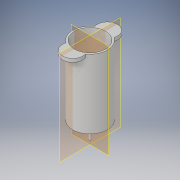
# Autodesk Inventor part: ReducedLargeSyrgine
Saved by Autodesk Inventor 2018 (Build 220112000, 112)
## iProperties
Created: 2020-03-29
Part Number: ReducedLargeSyrgine
Material: Generic
Document SubType Name: Modeling
Designer: Jesse R-B
Density: 1 g/cm^3
Appearance: Default
Author: Jesse R-B
Autodesk Inventor part; units mm, degrees
ref_plane "XZ Plane" through (0, 0, 0) normal (0, 1, 0) x (-1, 0, 0)
sketch "Sketch1" plane through (0, 0, 0) normal (0, 1, 0) x (-1, 0, 0)
  circle A0 centre (0, 0) radius 25.4
  dimension "d0" = 50.8
  constraints: 1 centre point, 1 coincident
  measures "d0" diameter of A0
extrude "Extrusion1" add sketch "Sketch1" along normal blind 101.6
sketch "Sketch2" plane through (0, 101.6, 0) normal (0, 1, 0) x (1, 0, 0)
  circle A0 centre (0, 0) radius 25.4 projected
  circle A1 centre (0, -25.4) radius 14.9225
  circle A2 centre (0, 25.4) radius 14.9225
  dimension "d3" = 29.845
  dimension "d4" = 29.845
  constraints: 2 centre point, 2 point on circle
  measures "d3" diameter of A1
  measures "d4" diameter of A2
extrude "Extrusion2" add sketch "Sketch2" against normal blind 5.08
sketch "Sketch3" plane through (0, 101.6, 0) normal (0, 1, 0) x (1, 0, 0)
  circle A0 centre (0, 0) radius 22.86
  dimension "d7" = 45.72
  constraints: 1 centre point, 1 coincident
  measures "d7" diameter of A0
extrude "Extrusion3" cut sketch "Sketch3" against normal blind 195.072
sketch "Sketch4" plane through (0, 0, 0) normal (0, -1, 0) x (1, 0, 0)
  circle A0 centre (0, 0) radius 2.921
  dimension "d10" = 5.842
  constraints: 1 centre point, 1 coincident
  measures "d10" diameter of A0
extrude "Extrusion4" add sketch "Sketch4" along normal blind 25.4 draft -4
sketch "Sketch5" plane through (0, 0, 0) normal (0, -1, 0) x (1, 0, 0)
  circle A0 centre (0, 0) radius 1.1449 projected
  circle A1 centre (0, 0) radius 22.86
  constraints: 1 centre point, 1 coincident
extrude "Extrusion5" add sketch "Sketch5" against normal blind 2.54
body "Solid1"
